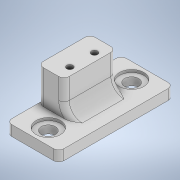
# Autodesk Inventor part: soporteendstop
Saved by Autodesk Inventor 2022 (Build 260153000, 153)
## iProperties
Created: 2022-03-17
Part Number: soporteendstop
Material: Genérico
Document SubType Name: Modeling
Designer: JK
Density: 1 g/cm^3
Appearance: Valor por defecto
Author: JK
Autodesk Inventor part; units mm, degrees
ref_plane "YZ Plane" through (0, 0, 0) normal (1, 0, 0) x (0, 1, 0)
ref_plane "XZ Plane" through (0, 0, 0) normal (0, 1, 0) x (-1, 0, 0)
ref_plane "XY Plane" through (0, 0, 0) normal (0, 0, 1) x (1, 0, 0)
sketch "Boceto1" plane through (0, 0, 0) normal (0, 1, 0) x (-1, 0, 0)
  line L0 (-10, 10) -> (10, 10)
  line L1 (10, 10) -> (10, -10)
  line L2 (10, -10) -> (-10, -10)
  line L3 (-10, -10) -> (-10, 10)
  line L4 (-10, 10) -> (10, -10) construction
  line L5 (10, 10) -> (-10, -10) construction
  line L6 (10, 22) -> (-10, 22)
  line L7 (-10, 22) -> (-10, -22)
  line L8 (-10, -22) -> (10, -22)
  line L9 (10, -22) -> (10, 22)
  circle A0 centre (0, 16) radius 2.7
  circle A1 centre (0, -16) radius 2.7
  point P0 (0, 0)
  dimension "d0" = 20
  dimension "d1" = 20
  dimension "d2" = 5.4
  dimension "d3" = 5.4
  dimension "d4" = 6
  dimension "d5" = 6
  dimension "d6" = 6
  dimension "d7" = 6
  constraints: 20 end point, 4 parallel, 2 centre point, 2 collinear, 2 horizontal, 2 midpoint, 2 perpendicular
  measures "d0" distance between parallel lines of L1 L3
  measures "d1" distance of L0.end L1.end
  measures "d2" diameter of A0
  measures "d3" diameter of A1
  measures "d4" distance from line of L0 A0.centre
  measures "d5" distance from line of L2 A1.centre
  measures "d6" distance from line of L8 A1.centre
  measures "d7" distance from line of L6 A0.centre
extrude "Extrusión1" add sketch "Boceto1" along normal blind 17
sketch "Boceto2" plane through (0, 17, 0) normal (0, 1, 0) x (1, 0, 0)
  circle A0 centre (-3, -4.75) radius 1.2
  circle A1 centre (-3, 4.75) radius 1.2
  line L0 (-10, 22) -> (-10, -22) projected
  point P0 (0, 0)
  dimension "d10" = 2.4
  dimension "d11" = 9.5
  dimension "d12" = 4.75
  dimension "d13" = 7
  constraints: 2 centre point, 1 equal radius, 1 vertical alignment
  measures "d10" diameter of A0
  measures "d11" distance of A1.centre A0.centre
  measures "d12" vertical distance of A1.centre point (0, 0)
  measures "d13" distance from line of L0 A0.centre
extrude "Extrusión2" cut sketch "Boceto2" against normal through all
sketch "Boceto3" plane through (0, 17, 0) normal (0, 1, 0) x (1, 0, 0)
  line L0 (-10, 22) -> (-10, -22) projected
  line L1 (10, -10) -> (-10, -10)
  line L2 (-10, -10) -> (-10, 10)
  line L3 (-10, 10) -> (10, 10)
  line L4 (10, 10) -> (10, -10)
  line L5 (10, -10) -> (-10, 10) construction
  line L6 (-10, -10) -> (10, 10) construction
  circle A0 centre (-3, 4.75) radius 1.2 projected
  circle A1 centre (-3, -4.75) radius 1.2 projected
  line L7 (10, -22) -> (10, 22) projected
  line L8 (10, 22) -> (-10, 22) projected
  line L9 (-10, 22) -> (-10, -22) projected
  line L10 (-10, -22) -> (10, -22) projected
  circle A2 centre (0, -16) radius 2.7 projected
  circle A3 centre (0, 16) radius 2.7 projected
  point P0 (0, 0)
  point P1 (-10, -22)
  point P2 (-10, -10)
  dimension "d16" = 20
  constraints: 12 end point, 2 midpoint, 2 parallel, 1 horizontal, 1 perpendicular, 1 point on line
  measures "d16" distance between parallel lines of L3 L1
extrude "Extrusión3" cut sketch "Boceto3" against normal blind 13 contours L8 L7 L3 L0 | L1 L7 L10 L0
sketch "Boceto4" plane through (0, 4, 0) normal (0, 1, 0) x (1, 0, 0)
  circle A0 centre (0, -16) radius 2.7 projected
  circle A1 centre (0, -16) radius 4.7
  circle A2 centre (0, 16) radius 2.7 projected
  circle A3 centre (0, 16) radius 4.7
  point P0 (0, 0)
  dimension "d19" = 9.4
  constraints: 2 centre point, 2 coincident, 1 equal radius
  measures "d19" diameter of A1
extrude "Extrusión4" cut sketch "Boceto4" against normal blind 1
sketch "Boceto5" plane through (0, 17, 0) normal (0, 1, 0) x (1, 0, 0)
  line L0 (-10, -10) -> (10, -10) projected
  line L1 (10, 10) -> (-10, 10) projected
  line L2 (10, -10) -> (0, -10)
  line L3 (0, -10) -> (0, 10)
  line L4 (0, 10) -> (10, 10)
  line L5 (10, 10) -> (10, -10)
  point P0 (0, 0)
  point P1 (0, -10)
  dimension "d22" = 10
  constraints: 8 end point, 2 parallel, 1 horizontal, 1 midpoint, 1 perpendicular
  measures "d22" distance between parallel lines of L5 L3
extrude "Extrusión5" cut sketch "Boceto5" against normal up to surface (13 mm away)
fillet "Empalme1" radius 2 4 edges at (10, 2, 22) (-10, 2, 22) (10, 2, -22) (-10, 2, -22)
fillet "Empalme2" radius 5 1 edges at (0, 4, 0)
fillet "Empalme3" radius 2 6 edges at (-10, 10.5, 10) (-10, 10.5, -10) (0, 13, 10) (0, 13, -10) (1.4645, 5.4645, -10) (1.4645, 5.4645, 10)
sketch "Boceto6" plane through (0, 0, 0) normal (0, -1, 0) x (1, 0, 0)
  circle A0 centre (-3, -4.75) radius 1.2 projected
  circle A1 centre (-3, -4.75) radius 2.15
  circle A2 centre (-3, 4.75) radius 1.2 projected
  circle A3 centre (-3, 4.75) radius 2.15
  line L0 (-5.4826, -4.75) -> (-4.2413, -2.6)
  line L1 (-4.2413, -2.6) -> (-1.7587, -2.6)
  line L2 (-1.7587, -2.6) -> (-0.5174, -4.75)
  line L3 (-0.5174, -4.75) -> (-1.7587, -6.9)
  line L4 (-1.7587, -6.9) -> (-4.2413, -6.9)
  line L5 (-4.2413, -6.9) -> (-5.4826, -4.75)
  line L6 (-5.4826, 4.75) -> (-4.2413, 6.9)
  line L7 (-4.2413, 6.9) -> (-1.7587, 6.9)
  line L8 (-1.7587, 6.9) -> (-0.5174, 4.75)
  line L9 (-0.5174, 4.75) -> (-1.7587, 2.6)
  line L10 (-1.7587, 2.6) -> (-4.2413, 2.6)
  line L11 (-4.2413, 2.6) -> (-5.4826, 4.75)
  point P0 (0, 0)
  dimension "d29" = 4.3
  dimension "d30" = 4.3
  constraints: 24 end point, 4 coincident, 2 centre point, 2 horizontal, 2 tangent, 26 other
  measures "d29" diameter of A1
  measures "d30" diameter of A3
extrude "Extrusión6" cut sketch "Boceto6" against normal blind 15 contours A0 | A1 | A1 L2 L3 | A1 L1 L2 | L3 L4 A1 | A1 L0 L1 | L4 L5 A1 | A1 L5 L0 | A2 | A3 | A3 L8 L9 | A3 L7 L8 | L9 L10 A3 | A3 L6 L7 | L10 L11 A3 | A3 L11 L6
